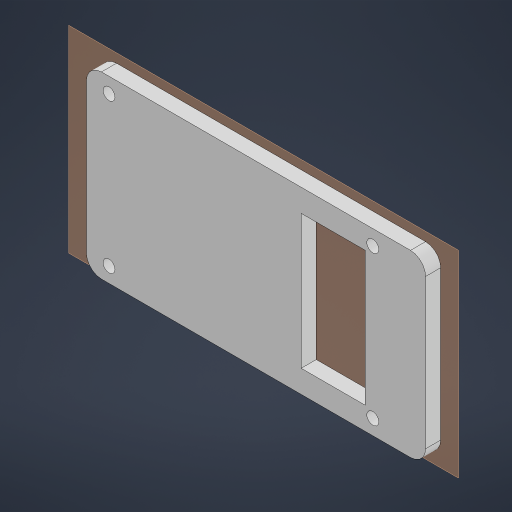
# Autodesk Inventor part: STlink_Top
Saved by Autodesk Inventor 2024.2 (Build 282272000, 272)
## iProperties
Created: 2024-03-15
Part Number: STlink_Top
Material: 一般
Document SubType Name: Modeling
Designer: Hanaoka
Density: 1 g/cm^3
Appearance: 既定
Author: Hanaoka
Autodesk Inventor part; units mm, degrees
ref_plane "YZ Plane" through (0, 0, 0) normal (1, 0, 0) x (0, 1, 0)
ref_plane "XZ Plane" through (0, 0, 0) normal (0, 1, 0) x (-1, 0, 0)
ref_plane "XY Plane" through (0, 0, 0) normal (0, 0, 1) x (1, 0, 0)
ref_plane "作業平面1" through (0, 0, 0) normal (0, 0, 1) x (1, 0, 0)
sketch "スケッチ1" plane through (0, 0, 0) normal (0, 0, 1) x (1, 0, 0)
  circle A0 centre (16.5, -9.9) radius 0.8 projected
  circle A1 centre (-18.5, 9.9) radius 0.8 projected
  circle A2 centre (16.5, 9.9) radius 0.8 projected
  circle A3 centre (-18.5, -9.9) radius 0.8 projected
  arc A4 (-21.5, -7.9) -> (-23.5, -9.9) centre (-21.5, -9.9) ccw projected
  line L0 (-23.5, -9.9) -> (-23.5, -11.9) projected
  line L1 (-23.5, -11.9) -> (23.5, -11.9) projected
  line L2 (23.5, -11.9) -> (23.5, 11.9) projected
  line L3 (23.5, 11.9) -> (-23.5, 11.9) projected
  line L4 (-23.5, 11.9) -> (-23.5, 9.9) projected
  arc A5 (-23.5, 9.9) -> (-21.5, 7.9) centre (-21.5, 9.9) ccw projected
  line L5 (-21.5, 7.9) -> (21.5, 7.9) projected
  line L6 (21.5, 7.9) -> (21.5, -7.9) projected
  line L7 (21.5, -7.9) -> (-21.5, -7.9) projected
  line L8 (-21.5, 11.9) -> (-21.5, -11.9)
  point P0 (0, 0)
  constraints: 4 point on line, 2 end point
ref_plane "作業平面2" through (0, 0, 0) normal (0, 0, 1) x (1, 0, 0)
extrude "押し出し1" add sketch "スケッチ1" along normal blind 2 contours L8 L5 L6 L7 | L7 L6 L5 L8 L3 L2 L1
fillet "フィレット1" radius 2 4 edges at (23.5, 11.9, 1) (23.5, -11.9, 1) (-21.5, -11.9, 1) (-21.5, 11.9, 1)
sketch "スケッチ2" plane through (0, 0, 2) normal (0, 0, 1) x (1, 0, 0)
  line L0 (15.5, 8.9) -> (7, 8.9)
  line L1 (7, 8.9) -> (7, -8.9)
  line L2 (7, -8.9) -> (15.5, -8.9)
  line L3 (15.5, -8.9) -> (15.5, 8.9)
  circle A0 centre (16.5, 9.9) radius 0.8 projected
  circle A1 centre (16.5, -9.9) radius 0.8 projected
  point P0 (0, 0)
  dimension "d3" = 1
  dimension "d4" = 8.5
  dimension "d5" = 1
  dimension "d6" = 1
  constraints: 8 end point, 2 parallel, 1 horizontal, 1 perpendicular
  measures "d3" horizontal distance of A0.centre L0.start
  measures "d4" distance of L0.start L0.end
  measures "d5" horizontal distance of A0.centre L0.start
  measures "d6" horizontal distance of A1.centre L2.end
extrude "押し出し2" cut sketch "スケッチ2" against normal up to surface (2 mm away) contours L3 L2 L1 L0
